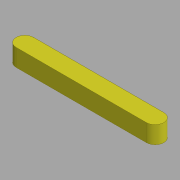
# Autodesk Inventor part: LED yellow
Saved by Autodesk Inventor 2014 SP2 (Build 180246200, 246)
## iProperties
Created: 2016-01-21
Part Number: LED yellow
Material: ABS plast
Document SubType Name: Modeling
Designer: Mervart
Mass: 0.0702602 g
Surface Area: 1.3885 cm^2
Volume: 0.0662832 cm^3
Density: 1.06 g/cm^3
Appearance: Kanárková
LastSaveDate: 21.09.2010
Hmotnost: 0
Author: Mervart
Autodesk Inventor part; units mm, degrees
ref_plane "YZ Plane" through (0, 0, 0) normal (1, 0, 0) x (0, 1, 0)
ref_plane "XZ Plane" through (0, 0, 0) normal (0, 1, 0) x (-1, 0, 0)
ref_plane "XY Plane" through (0, 0, 0) normal (0, 0, 1) x (1, 0, 0)
sketch "Náčrt4" plane through (0, 0, 0) normal (0, 0, 1) x (1, 0, 0)
  line L0 (-27.9693, -0.2458) -> (-12.9693, -0.2458) construction
  line L1 (-12.9693, -2.2458) -> (-27.9693, -2.2458) construction
  line L2 (-45.9693, -0.2458) -> (-30.9693, -0.2458) construction
  line L3 (-30.9693, -2.2458) -> (-45.9693, -2.2458) construction
  line L4 (-63.9693, -0.2458) -> (-48.9693, -0.2458) construction
  line L5 (-48.9693, -2.2458) -> (-63.9693, -2.2458) construction
  line L6 (-63.9693, 13.2542) -> (-4.8293, 13.2542) construction
  arc A0 (-63.9693, 13.2542) -> (-73.2693, 3.9542) centre (-63.9693, 3.9542) ccw construction
  line L7 (-73.2693, -86.0458) -> (-73.2693, 3.9542) construction
  arc A1 (-73.2693, -86.0458) -> (-63.9693, -95.3458) centre (-63.9693, -86.0458) ccw construction
  line L8 (-1.9693, -95.3458) -> (-63.9693, -95.3458) construction
  line L9 (-1.9693, -95.3458) -> (-1.9693, -1.0458) construction
  line L10 (-1.9693, -1.0458) -> (-4.8293, 13.2542) construction
  line L11 (-64.9693, -20.2458) -> (-64.9693, -6.2458) construction
  line L12 (-63.4693, -4.7458) -> (-49.4693, -4.7458) construction
  line L13 (-47.9693, -6.2458) -> (-47.9693, -20.2458) construction
  line L14 (-49.4693, -21.7458) -> (-63.4693, -21.7458) construction
  circle A2 centre (-38.4592, 9.4542) radius 0.3 construction
  circle A3 centre (-34.9592, 5.9542) radius 0.3 construction
  circle A4 centre (-38.4592, 2.4542) radius 0.3 construction
  circle A5 centre (-41.9592, 5.9542) radius 0.3 construction
  circle A6 centre (-38.4592, 5.9542) radius 0.3 construction
  circle A7 centre (-40.9341, 8.4291) radius 0.3 construction
  circle A8 centre (-40.9341, 3.4794) radius 0.3 construction
  circle A9 centre (-35.9844, 3.4794) radius 0.3 construction
  circle A10 centre (-35.9844, 8.4291) radius 0.3 construction
  line L15 (-45.9693, -0.2458) -> (-30.9693, -0.2458)
  line L16 (-30.9693, -2.2458) -> (-45.9693, -2.2458)
  line L17 (-33.7677, -85.5406) -> (-34.3413, -86.3597) projected
  arc A11 (-34.3413, -86.3597) -> (-42.5973, -86.3597) centre (-38.4693, -92.2551) ccw projected
  line L18 (-42.5973, -86.3597) -> (-43.1709, -85.5406) projected
  arc A12 (-33.7677, -85.5406) -> (-43.1709, -85.5406) centre (-38.4693, -92.2551) ccw projected
  circle A13 centre (-38.4693, -92.2551) radius 0.9 projected
  line L19 (-35.9457, -88.0585) -> (-36.5193, -88.8776) projected
  arc A14 (-36.5193, -88.8776) -> (-40.4193, -88.8776) centre (-38.4693, -92.2551) ccw projected
  line L20 (-40.4193, -88.8776) -> (-40.9929, -88.0585) projected
  arc A15 (-35.9457, -88.0585) -> (-40.9929, -88.0585) centre (-38.4693, -92.2551) ccw projected
  arc A16 (-31.8749, -82.8374) -> (-45.0637, -82.8374) centre (-38.4693, -92.2551) ccw projected
  line L21 (-31.8749, -82.8374) -> (-32.4485, -83.6565) projected
  arc A17 (-32.4485, -83.6565) -> (-44.4901, -83.6565) centre (-38.4693, -92.2551) ccw projected
  line L22 (-44.4901, -83.6565) -> (-45.0637, -82.8374) projected
  line L23 (-28.9693, -74.2458) -> (-28.9693, -60.2458) projected
  arc A18 (-27.4693, -58.7458) -> (-28.9693, -60.2458) centre (-27.4693, -60.2458) ccw projected
  line L24 (-27.4693, -58.7458) -> (-13.4693, -58.7458) projected
  arc A19 (-11.9693, -60.2458) -> (-13.4693, -58.7458) centre (-13.4693, -60.2458) ccw projected
  line L25 (-11.9693, -60.2458) -> (-11.9693, -74.2458) projected
  arc A20 (-13.4693, -75.7458) -> (-11.9693, -74.2458) centre (-13.4693, -74.2458) ccw projected
  line L26 (-13.4693, -75.7458) -> (-27.4693, -75.7458) projected
  arc A21 (-28.9693, -74.2458) -> (-27.4693, -75.7458) centre (-27.4693, -74.2458) ccw projected
  line L27 (-46.9693, -74.2458) -> (-46.9693, -60.2458) projected
  arc A22 (-45.4693, -58.7458) -> (-46.9693, -60.2458) centre (-45.4693, -60.2458) ccw projected
  line L28 (-45.4693, -58.7458) -> (-31.4693, -58.7458) projected
  arc A23 (-29.9693, -60.2458) -> (-31.4693, -58.7458) centre (-31.4693, -60.2458) ccw projected
  line L29 (-29.9693, -60.2458) -> (-29.9693, -74.2458) projected
  arc A24 (-31.4693, -75.7458) -> (-29.9693, -74.2458) centre (-31.4693, -74.2458) ccw projected
  line L30 (-31.4693, -75.7458) -> (-45.4693, -75.7458) projected
  arc A25 (-46.9693, -74.2458) -> (-45.4693, -75.7458) centre (-45.4693, -74.2458) ccw projected
  line L31 (-64.9693, -74.2458) -> (-64.9693, -60.2458) projected
  arc A26 (-63.4693, -58.7458) -> (-64.9693, -60.2458) centre (-63.4693, -60.2458) ccw projected
  line L32 (-63.4693, -58.7458) -> (-49.4693, -58.7458) projected
  arc A27 (-47.9693, -60.2458) -> (-49.4693, -58.7458) centre (-49.4693, -60.2458) ccw projected
  line L33 (-47.9693, -60.2458) -> (-47.9693, -74.2458) projected
  arc A28 (-49.4693, -75.7458) -> (-47.9693, -74.2458) centre (-49.4693, -74.2458) ccw projected
  line L34 (-49.4693, -75.7458) -> (-63.4693, -75.7458) projected
  arc A29 (-64.9693, -74.2458) -> (-63.4693, -75.7458) centre (-63.4693, -74.2458) ccw projected
  line L35 (-28.9693, -56.2458) -> (-28.9693, -42.2458) projected
  arc A30 (-27.4693, -40.7458) -> (-28.9693, -42.2458) centre (-27.4693, -42.2458) ccw projected
  line L36 (-27.4693, -40.7458) -> (-13.4693, -40.7458) projected
  arc A31 (-11.9693, -42.2458) -> (-13.4693, -40.7458) centre (-13.4693, -42.2458) ccw projected
  line L37 (-11.9693, -42.2458) -> (-11.9693, -56.2458) projected
  arc A32 (-13.4693, -57.7458) -> (-11.9693, -56.2458) centre (-13.4693, -56.2458) ccw projected
  line L38 (-13.4693, -57.7458) -> (-27.4693, -57.7458) projected
  arc A33 (-28.9693, -56.2458) -> (-27.4693, -57.7458) centre (-27.4693, -56.2458) ccw projected
  line L39 (-46.9693, -56.2458) -> (-46.9693, -42.2458) projected
  arc A34 (-45.4693, -40.7458) -> (-46.9693, -42.2458) centre (-45.4693, -42.2458) ccw projected
  line L40 (-45.4693, -40.7458) -> (-31.4693, -40.7458) projected
  arc A35 (-29.9693, -42.2458) -> (-31.4693, -40.7458) centre (-31.4693, -42.2458) ccw projected
  line L41 (-29.9693, -42.2458) -> (-29.9693, -56.2458) projected
  arc A36 (-31.4693, -57.7458) -> (-29.9693, -56.2458) centre (-31.4693, -56.2458) ccw projected
  line L42 (-31.4693, -57.7458) -> (-45.4693, -57.7458) projected
  arc A37 (-46.9693, -56.2458) -> (-45.4693, -57.7458) centre (-45.4693, -56.2458) ccw projected
  line L43 (-64.9693, -56.2458) -> (-64.9693, -42.2458) projected
  arc A38 (-63.4693, -40.7458) -> (-64.9693, -42.2458) centre (-63.4693, -42.2458) ccw projected
  line L44 (-63.4693, -40.7458) -> (-49.4693, -40.7458) projected
  arc A39 (-47.9693, -42.2458) -> (-49.4693, -40.7458) centre (-49.4693, -42.2458) ccw projected
  line L45 (-47.9693, -42.2458) -> (-47.9693, -56.2458) projected
  arc A40 (-49.4693, -57.7458) -> (-47.9693, -56.2458) centre (-49.4693, -56.2458) ccw projected
  line L46 (-49.4693, -57.7458) -> (-63.4693, -57.7458) projected
  arc A41 (-64.9693, -56.2458) -> (-63.4693, -57.7458) centre (-63.4693, -56.2458) ccw projected
  line L47 (-28.9693, -38.2458) -> (-28.9693, -24.2458) projected
  arc A42 (-27.4693, -22.7458) -> (-28.9693, -24.2458) centre (-27.4693, -24.2458) ccw projected
  line L48 (-27.4693, -22.7458) -> (-13.4693, -22.7458) projected
  arc A43 (-11.9693, -24.2458) -> (-13.4693, -22.7458) centre (-13.4693, -24.2458) ccw projected
  line L49 (-11.9693, -24.2458) -> (-11.9693, -38.2458) projected
  arc A44 (-13.4693, -39.7458) -> (-11.9693, -38.2458) centre (-13.4693, -38.2458) ccw projected
  line L50 (-13.4693, -39.7458) -> (-27.4693, -39.7458) projected
  arc A45 (-28.9693, -38.2458) -> (-27.4693, -39.7458) centre (-27.4693, -38.2458) ccw projected
  line L51 (-46.9693, -38.2458) -> (-46.9693, -24.2458) projected
  arc A46 (-45.4693, -22.7458) -> (-46.9693, -24.2458) centre (-45.4693, -24.2458) ccw projected
  line L52 (-45.4693, -22.7458) -> (-31.4693, -22.7458) projected
  arc A47 (-29.9693, -24.2458) -> (-31.4693, -22.7458) centre (-31.4693, -24.2458) ccw projected
  line L53 (-29.9693, -24.2458) -> (-29.9693, -38.2458) projected
  arc A48 (-31.4693, -39.7458) -> (-29.9693, -38.2458) centre (-31.4693, -38.2458) ccw projected
  line L54 (-31.4693, -39.7458) -> (-45.4693, -39.7458) projected
  arc A49 (-46.9693, -38.2458) -> (-45.4693, -39.7458) centre (-45.4693, -38.2458) ccw projected
  line L55 (-64.9693, -38.2458) -> (-64.9693, -24.2458) projected
  arc A50 (-63.4693, -22.7458) -> (-64.9693, -24.2458) centre (-63.4693, -24.2458) ccw projected
  line L56 (-63.4693, -22.7458) -> (-49.4693, -22.7458) projected
  arc A51 (-47.9693, -24.2458) -> (-49.4693, -22.7458) centre (-49.4693, -24.2458) ccw projected
  line L57 (-47.9693, -24.2458) -> (-47.9693, -38.2458) projected
  arc A52 (-49.4693, -39.7458) -> (-47.9693, -38.2458) centre (-49.4693, -38.2458) ccw projected
  line L58 (-49.4693, -39.7458) -> (-63.4693, -39.7458) projected
  arc A53 (-64.9693, -38.2458) -> (-63.4693, -39.7458) centre (-63.4693, -38.2458) ccw projected
  line L59 (-28.9693, -20.2458) -> (-28.9693, -6.2458) projected
  arc A54 (-27.4693, -4.7458) -> (-28.9693, -6.2458) centre (-27.4693, -6.2458) ccw projected
  line L60 (-27.4693, -4.7458) -> (-13.4693, -4.7458) projected
  arc A55 (-11.9693, -6.2458) -> (-13.4693, -4.7458) centre (-13.4693, -6.2458) ccw projected
  line L61 (-11.9693, -6.2458) -> (-11.9693, -20.2458) projected
  arc A56 (-13.4693, -21.7458) -> (-11.9693, -20.2458) centre (-13.4693, -20.2458) ccw projected
  line L62 (-13.4693, -21.7458) -> (-27.4693, -21.7458) projected
  arc A57 (-28.9693, -20.2458) -> (-27.4693, -21.7458) centre (-27.4693, -20.2458) ccw projected
  line L63 (-46.9693, -20.2458) -> (-46.9693, -6.2458) projected
  arc A58 (-45.4693, -4.7458) -> (-46.9693, -6.2458) centre (-45.4693, -6.2458) ccw projected
  line L64 (-45.4693, -4.7458) -> (-31.4693, -4.7458) projected
  arc A59 (-29.9693, -6.2458) -> (-31.4693, -4.7458) centre (-31.4693, -6.2458) ccw projected
  line L65 (-29.9693, -6.2458) -> (-29.9693, -20.2458) projected
  arc A60 (-31.4693, -21.7458) -> (-29.9693, -20.2458) centre (-31.4693, -20.2458) ccw projected
  line L66 (-31.4693, -21.7458) -> (-45.4693, -21.7458) projected
  arc A61 (-46.9693, -20.2458) -> (-45.4693, -21.7458) centre (-45.4693, -20.2458) ccw projected
  arc A62 (-27.9693, -0.2458) -> (-27.9693, -2.2458) centre (-27.9693, -1.2458) ccw projected
  arc A63 (-12.9693, -2.2458) -> (-12.9693, -0.2458) centre (-12.9693, -1.2458) ccw projected
  arc A64 (-45.9693, -0.2458) -> (-45.9693, -2.2458) centre (-45.9693, -1.2458) ccw projected
  arc A65 (-30.9693, -2.2458) -> (-30.9693, -0.2458) centre (-30.9693, -1.2458) ccw projected
  arc A66 (-63.9693, -0.2458) -> (-63.9693, -2.2458) centre (-63.9693, -1.2458) ccw projected
  arc A67 (-48.9693, -2.2458) -> (-48.9693, -0.2458) centre (-48.9693, -1.2458) ccw projected
  arc A68 (-63.4693, -4.7458) -> (-64.9693, -6.2458) centre (-63.4693, -6.2458) ccw projected
  arc A69 (-47.9693, -6.2458) -> (-49.4693, -4.7458) centre (-49.4693, -6.2458) ccw projected
  arc A70 (-49.4693, -21.7458) -> (-47.9693, -20.2458) centre (-49.4693, -20.2458) ccw projected
  arc A71 (-64.9693, -20.2458) -> (-63.4693, -21.7458) centre (-63.4693, -20.2458) ccw projected
  point P0 (0, 0)
  point P1 (-29.9693, -1.2458)
  constraints: 5 point on circle, 4 end point, 1 horizontal, 1 parallel
extrude "Vysunutí1" add sketch "Náčrt4" against normal blind 2 contours L15 A65 L16 A64
